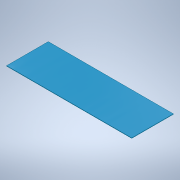
# Autodesk Inventor part: Model2
Saved by Autodesk Inventor 2020.3 (Build 243373000, 373)
## iProperties
Created: 2021-04-22
Part Number: Model2
Material: Generic
Document SubType Name: Modeling
Designer: alexo
Density: 1 g/cm^3
Appearance: Sky Blue Dark
Author: alexo
Autodesk Inventor part; units mm, degrees
ref_plane "YZ Plane" through (0, 0, 0) normal (1, 0, 0) x (0, 1, 0)
ref_plane "XZ Plane" through (0, 0, 0) normal (0, 1, 0) x (-1, 0, 0)
ref_plane "XY Plane" through (0, 0, 0) normal (0, 0, 1) x (1, 0, 0)
sketch "Sketch1" plane through (0, 0, 0) normal (0, 1, 0) x (-1, 0, 0)
  line L0 (-78, -26) -> (78, -26)
  line L1 (78, -26) -> (78, 26)
  line L2 (78, 26) -> (-78, 26)
  line L3 (-78, 26) -> (-78, -26)
  line L4 (-78, -26) -> (78, 26) construction
  line L5 (78, -26) -> (-78, 26) construction
  point P0 (0, 0)
  dimension "d0" = 52
  dimension "d1" = 156
  constraints: 12 end point, 2 midpoint, 2 parallel, 1 horizontal, 1 perpendicular
  measures "d0" distance of L0.end L1.end
  measures "d1" distance of L1.end L2.end
extrude "Extrusion1" add sketch "Sketch1" along normal blind 0.5
body "Solid1"
